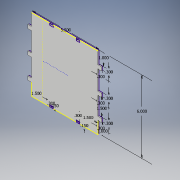
# Autodesk Inventor part: BB Gun Back Panel
Saved by Autodesk Inventor 2018 (Build 220112000, 112)
## iProperties
Created: 2019-05-24
Part Number: BB Gun Back Panel
Material: Generic
Document SubType Name: Modeling
Designer: 871357
Density: 1 g/cm^3
Appearance: Default
Author: 871357
Autodesk Inventor part; units mm, degrees
ref_plane "YZ Plane" through (0, 0, 0) normal (1, 0, 0) x (0, 1, 0)
ref_plane "XZ Plane" through (0, 0, 0) normal (0, 1, 0) x (-1, 0, 0)
ref_plane "XY Plane" through (0, 0, 0) normal (0, 0, 1) x (1, 0, 0)
sketch "Sketch1" plane through (0, 0, 0) normal (0, 0, 1) x (1, 0, 0)
  line L0 (0, 0) -> (139.7, 0)
  line L1 (139.7, 0) -> (139.7, 152.4)
  line L2 (139.7, 152.4) -> (0, 152.4)
  line L3 (139.7, 127) -> (147.32, 127)
  line L4 (147.32, 127) -> (147.32, 119.38)
  line L5 (147.32, 119.38) -> (139.7, 119.38)
  line L6 (139.7, 119.38) -> (139.7, 127)
  line L7 (139.7, 78.74) -> (147.32, 78.74)
  line L8 (147.32, 78.74) -> (147.32, 71.12)
  line L9 (147.32, 71.12) -> (139.7, 71.12)
  line L10 (139.7, 71.12) -> (139.7, 78.74)
  line L11 (139.7, 33.02) -> (147.32, 33.02)
  line L12 (147.32, 33.02) -> (147.32, 25.4)
  line L13 (147.32, 25.4) -> (139.7, 25.4)
  line L14 (139.7, 25.4) -> (139.7, 33.02)
  line L15 (69.85, 152.4) -> (69.85, 0) construction
  line L16 (0, 127) -> (-7.62, 127)
  line L17 (-7.62, 127) -> (-7.62, 119.38)
  line L18 (-7.62, 119.38) -> (0, 119.38)
  line L19 (0, 78.74) -> (-7.62, 78.74)
  line L20 (-7.62, 78.74) -> (-7.62, 71.12)
  line L21 (-7.62, 71.12) -> (0, 71.12)
  line L22 (0, 33.02) -> (-7.62, 33.02)
  line L23 (-7.62, 33.02) -> (-7.62, 25.4)
  line L24 (-7.62, 25.4) -> (0, 25.4)
  line L25 (0, 152.4) -> (0, 127)
  line L26 (0, 119.38) -> (0, 78.74)
  line L27 (0, 71.12) -> (0, 33.02)
  line L28 (0, 25.4) -> (0, 0)
  dimension "d0" = 139.7
  dimension "d1" = 152.4
  dimension "d2" = 7.62
  dimension "d3" = 7.62
  dimension "d4" = 25.4
  dimension "d5" = 7.62
  dimension "d6" = 7.62
  dimension "d7" = 7.62
  dimension "d8" = 7.62
  dimension "d9" = 25.4
  dimension "d10" = 38.1
  constraints: 58 end point, 12 symmetric about line, 11 parallel, 4 horizontal, 4 perpendicular, 3 point on line, 2 midpoint
  measures "d0" distance of L2.end L1.end
  measures "d1" distance of L0.end L1.end
  measures "d2" distance of L4.end L5.end
  measures "d3" distance of L3.end L4.end
  measures "d4" distance between parallel lines of L2 L3
  measures "d5" distance of L8.end L9.end
  measures "d6" distance of L7.end L8.end
  measures "d7" distance of L12.end L13.end
  measures "d8" distance of L11.end L12.end
  measures "d9" distance between parallel lines of L0 L13
  measures "d10" distance between parallel lines of L9 L11
extrude "Extrusion1" add sketch "Sketch1" along normal blind 2.54
sketch "Sketch2" plane through (0, 0, 2.54) normal (0, 0, 1) x (1, 0, 0)
  line L0 (0, 0) -> (139.7, 0) projected
  line L1 (38.1, 0) -> (45.72, 0)
  line L2 (45.72, 0) -> (45.72, 3.81)
  line L3 (45.72, 3.81) -> (38.1, 3.81)
  line L4 (38.1, 3.81) -> (38.1, 0)
  line L5 (0, 25.4) -> (0, 0) projected
  line L6 (93.98, 0) -> (101.6, 0)
  line L7 (101.6, 0) -> (101.6, 3.81)
  line L8 (101.6, 3.81) -> (93.98, 3.81)
  line L9 (93.98, 3.81) -> (93.98, 0)
  line L10 (139.7, 0) -> (139.7, 25.4) projected
  line L11 (139.7, 152.4) -> (0, 152.4) projected
  line L12 (23.3559, 152.4) -> (23.3559, 0) construction
  line L13 (23.3559, 76.2) -> (77.5695, 76.2) construction
  line L14 (45.72, 152.4) -> (45.72, 148.59)
  line L15 (45.72, 148.59) -> (38.1, 148.59)
  line L16 (38.1, 148.59) -> (38.1, 152.4)
  line L17 (101.6, 152.4) -> (101.6, 148.59)
  line L18 (101.6, 148.59) -> (93.98, 148.59)
  line L19 (93.98, 148.59) -> (93.98, 152.4)
  line L20 (38.1, 152.4) -> (45.72, 152.4)
  line L21 (93.98, 152.4) -> (101.6, 152.4)
  dimension "d13" = 3.81
  dimension "d14" = 7.62
  dimension "d15" = 38.1
  dimension "d16" = 7.62
  dimension "d17" = 3.81
  dimension "d18" = 38.1
  constraints: 36 end point, 8 symmetric about line, 4 parallel, 4 point on line, 3 horizontal, 3 perpendicular, 2 collinear, 1 midpoint
  measures "d13" distance of L1.end L2.end
  measures "d14" distance of L2.end L3.end
  measures "d15" distance between parallel lines of L5 L4
  measures "d16" distance of L8.end L7.end
  measures "d17" distance of L7.end L6.end
  measures "d18" distance between parallel lines of L10 L7
extrude "Extrusion3" cut sketch "Sketch2" against normal blind 25.4
body "Solid1"
